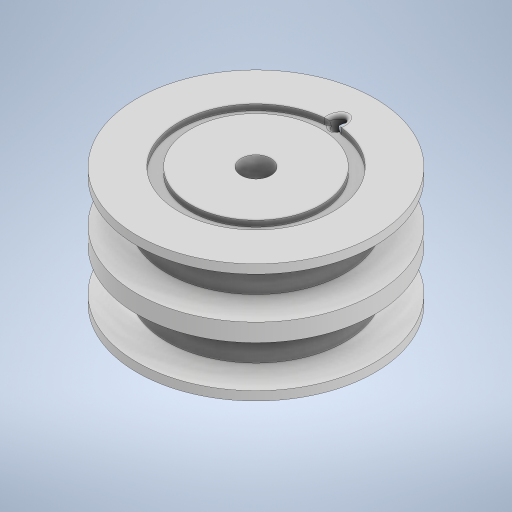
# Autodesk Inventor part: 커튼 휠
Saved by Autodesk Inventor 2023.1 (Build 271208000, 208)
## iProperties
Created: 2022-09-03
Part Number: 커튼 휠
Material: 일반
Document SubType Name: Modeling
Designer: fly01
Density: 1 g/cm^3
Appearance: 기본값
Author: fly01
Autodesk Inventor part; units mm, degrees
note: some values were not read from the file. Chosen so that the rebuilt part matches the saved one: arc direction of "돌출5".
ref_plane "YZ Plane" through (0, 0, 0) normal (1, 0, 0) x (0, 1, 0)
ref_plane "XZ Plane" through (0, 0, 0) normal (0, 1, 0) x (-1, 0, 0)
sketch "스케치1" plane through (0, 0, 0) normal (0, 1, 0) x (-1, 0, 0)
  circle A0 centre (0, 0) radius 4.5
  circle A1 centre (0, 0) radius 2.9
  line L0 (1.6279, -2.4) -> (-1.6279, -2.4)
  line L1 (0, -2.4) -> (0, -2.9) construction
  dimension "d0" = 9
  dimension "d1" = 5.8
  dimension "d2" = 0.5
  constraints: 4 end point, 3 point on circle, 2 centre point, 2 coincident, 1 horizontal, 1 midpoint, 1 vertical
  measures "d0" diameter of A0
  measures "d1" diameter of A1
  measures "d2" distance of L1.start L1.end
extrude "돌출1" add sketch "스케치1" along normal blind 6 contours A0 | L0 A1 picked at (-0.3384, -2.5055)
sketch "스케치2" plane through (0, 0, 0) normal (0, -1, 0) x (1, 0, 0)
  circle A0 centre (0, 0) radius 2.9
  constraints: 1 centre point, 1 coincident
extrude "돌출2" cut sketch "스케치2" against normal blind 1
sketch "스케치3" plane through (0, 6, 0) normal (0, 1, 0) x (1, 0, 0)
  circle A0 centre (0, 0) radius 4.5 projected
  circle A1 centre (0, 0) radius 1.5
  dimension "d7" = 3
  constraints: 1 centre point, 1 coincident
  measures "d7" diameter of A1
extrude "돌출3" add sketch "스케치3" against normal blind 2
sketch "스케치4" plane through (0, 6, 0) normal (0, 1, 0) x (1, 0, 0)
  circle A0 centre (0, 0) radius 2.5
  circle A1 centre (0, 0) radius 15
  dimension "d10" = 5
  dimension "d11" = 30
  constraints: 2 centre point, 2 coincident
  measures "d10" diameter of A0
  measures "d11" diameter of A1
sketch "스케치5" plane through (0, 0, 0) normal (0, 0, 1) x (1, 0, 0)
  line L0 (4.5, 6) -> (-4.5, 6) projected
  line L1 (0, 6) -> (20, 6)
  line L2 (20, 6) -> (20, 7.5)
  line L3 (20, 7.5) -> (15, 8)
  line L4 (15, 8) -> (15, 11)
  line L5 (15, 11) -> (0, 11) construction
  line L6 (0, 11) -> (0, 6)
  line L7 (0, 16) -> (20, 16)
  line L8 (20, 16) -> (20, 14.5)
  line L9 (20, 14.5) -> (15, 14)
  line L10 (15, 14) -> (15, 11)
  line L11 (0, 11) -> (0, 16)
  line L12 (1.5, 4) -> (1.5, 6) projected
  line L13 (1.5, 6) -> (1.5, 16)
  point P0 (0, 0)
  point P1 (4.5, 16)
  dimension "d12" = 5
  dimension "d13" = 3
  dimension "d14" = 1.5
  dimension "d15" = 5
  dimension "d16" = 20
  constraints: 24 end point, 5 symmetric about line, 4 perpendicular, 3 point on line, 1 horizontal, 1 midpoint, 1 parallel
  measures "d12" distance of L5.end L1.start
  measures "d13" distance of L3.end L4.end
  measures "d14" distance of L1.end L2.end
  measures "d15" distance between parallel lines of L2 L4
  measures "d16" distance of L1.start L1.end
revolve "회전1" add sketch "스케치5" angle 360 about axis through (0, 11, 0) along (0, 1, 0) contours L0 L13 L7 L8 L9 L10 L4 L3 L2 L1
sketch "스케치6" plane through (0, 0, 0) normal (1, 0, 0) x (0, 1, 0)
  line L0 (8, -15) -> (14, -15) projected
  line L1 (8, -15) -> (6, -13)
  line L2 (6, -20) -> (6, 20) projected
  line L3 (8, -15) -> (8, 15) projected
  line L4 (8, -15) -> (8.7898, -15.7898)
  line L5 (8.7898, -15.7898) -> (8.0827, -16.497)
  line L6 (8.0827, -16.497) -> (4.3816, -12.7959)
  line L7 (4.3816, -12.7959) -> (5.0888, -12.0888)
  line L8 (5.0888, -12.0888) -> (6, -13)
  point P0 (0, 0)
  dimension "d18" = 1
  dimension "d19" = 45
  constraints: 12 end point, 4 perpendicular, 2 point on line
  measures "d18" distance between parallel lines of L4 L6
  measures "d19" angle of L3 L1
revolve "회전2" cut sketch "스케치6" angle 360 about axis through (0, 8, -15) along (0, 0.7071068, -0.7071068)
mirror "미러1" about plane through (1.5, 16, 0) normal (0, 1, 0) of "회전1", "회전2"
sketch "스케치7" plane through (0, 26, 0) normal (0, 1, 0) x (1, 0, 0)
  circle A0 centre (0, 0) radius 2.5
  dimension "d21" = 5
  constraints: 1 centre point, 1 coincident
  measures "d21" diameter of A0
extrude "돌출4" cut sketch "스케치7" against normal blind 20
fillet "모깎기1" radius 3 1 edges at (4.5, 6, 0)
sketch "스케치8" plane through (0, 6, 0) normal (0, -1, 0) x (1, 0, 0)
  circle A0 centre (0, 0) radius 11
  ellipse E0 centre (0, -13) end of major axis (0, -14.4142) minor radius 1 projected
  circle A1 centre (0, 0) radius 13
  point P0 (0.9996, -12.9615)
  point P1 (-0.9996, -12.9615)
  dimension "d25" = 22
  constraints: 2 coincident, 1 centre point, 4 other
  measures "d25" diameter of A0
extrude "돌출5" cut sketch "스케치8" against normal blind 1 contours A1 E0 | E0 A1 picked at (0.1086, -12.5515) picked at (12.0932, -1.9453)
ref_plane "작업 평면1" through (0, 16, 0) normal (0, -1, 0) x (1, 0, 0)
mirror "미러2" about plane through (0, 16, 0) normal (0, -1, 0) of "돌출5"
fillet "모깎기3" radius 0.5 10 edges at (-0.7167, 26, -13.9863) (0.7167, 26, -13.9863) (0.9217, 25.4842, -12.9673) (-0.9217, 25.4842, -12.9673) (0, 25, -12.5858) (0.7167, 6, -13.9863) (-0.7167, 6, -13.9863) (0, 7, -12.5858) (0.9217, 6.5158, -12.9673) (-0.9217, 6.5158, -12.9673)
